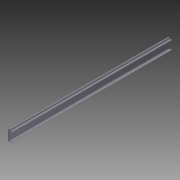
# Autodesk Inventor part: slide inner
Saved by Autodesk Inventor 2012 (Build 160160000, 160)
## iProperties
Created: 2011-12-02
Part Number: slide inner
Material: Steel
Document SubType Name: Modeling
Designer: Antonella
Density: 7.85 g/cm^3
Mass: 163.428 g
Surface Area: 532.739 cm^2
Volume: 20.8189 cm^3
Author: Antonella
Autodesk Inventor part; units mm, degrees
ref_plane "YZ Plane" through (0, 0, 0) normal (1, 0, 0) x (0, 1, 0)
ref_plane "XZ Plane" through (0, 0, 0) normal (0, 1, 0) x (-1, 0, 0)
ref_plane "XY Plane" through (0, 0, 0) normal (0, 0, 1) x (1, 0, 0)
sketch "Sketch1" plane through (0, 0, 0) normal (0, 0, 1) x (1, 0, 0)
  line L0 (-5.5563, 0) -> (11.1125, 0) projected
  line L1 (0, -22.225) -> (0, 22.225) projected
  line L2 (8.7313, 12.7) -> (3.175, 12.7)
  line L3 (3.175, 12.7) -> (3.175, -12.7) construction
  line L4 (3.175, -12.7) -> (8.7313, -12.7)
  line L5 (-3.175, 12.7) -> (-3.175, -12.7)
  arc A0 (3.175, 12.7) -> (-3.175, 12.7) centre (0, 12.7) ccw
  arc A1 (-3.175, -12.7) -> (3.175, -12.7) centre (0, -12.7) ccw
  line L6 (8.7313, 12.7) -> (8.7313, -12.7) construction
  arc A2 (2.3812, 12.7) -> (-2.3812, 12.7) centre (0, 12.7) ccw
  line L7 (-2.3812, 12.7) -> (-2.3812, -12.7)
  arc A3 (-2.3812, -12.7) -> (2.3812, -12.7) centre (0, -12.7) ccw
  line L8 (8.7313, -11.9062) -> (2.3812, -11.9062)
  line L9 (8.7313, 11.9062) -> (2.3812, 11.9062)
  line L10 (8.7313, -12.7) -> (8.7313, -11.9062)
  line L11 (8.7313, 11.9062) -> (8.7313, 12.7)
  line L12 (2.3812, 11.9062) -> (2.3812, 12.7)
  line L13 (2.3812, -12.7) -> (2.3812, -11.9062)
  point P0 (0, 0)
  point P1 (3.175, 0)
  point P2 (-3.175, 0)
  dimension "d0" = 25.4
  dimension "d1" = 11.9062
  dimension "d2" = 25.4
  dimension "d3" = 5.5563
  dimension "d4" = 0.7937
  dimension "d5" = 0.7937
  constraints: 24 end point, 11 perpendicular, 8 point on circle, 4 centre point, 4 equal length, 4 tangent, 2 horizontal alignment, 2 midpoint, 2 point on line, 1 vertical alignment, 2 other
  measures "d0" distance between parallel lines of L4 L2
  measures "d1" distance between parallel lines of L5 L6
  measures "d2" distance of L5.start L5.end
  measures "d3" distance of L3.end L4.end
  measures "d4" distance between parallel lines of L4 L8
  measures "d5" distance between parallel lines of L5 L7
extrude "Extrusion1" add sketch "Sketch1" along normal blind 457.2 contours L5 A0 L1 A2 L7 L0 | L0 L7 A3 L1 A1 L5 | A0 L2 L11 L9 L12 A2 L1 | L1 A3 L13 L8 L10 L4 A1
body "Solid1"
